00ed2536-3d80-4f07-8851-4f49f1606498 (Autodesk Fusion 360 design; units mm, degrees)
Autodesk Fusion 360 part; units mm, degrees
sketch "Sketch1" plane through (0, 0, 0) normal (0, 0, 1) x (1, 0, 0)
  circle A0 centre (0, 0) radius 7.9375
  circle A1 centre (0, 0) radius 11.1125
  dimension "d1" = 15.875
  dimension "d2" = 22.225
  measures "d1" diameter of A0
  measures "d2" diameter of A1
extrude "Extrude1" add sketch "Sketch1" along normal blind 31.75
sketch "Sketch2" plane through (0, 0, 0) normal (0, 0, -1) x (-1, 0, 0)
  circle A0 centre (0, 0) radius 11.1125
  circle A1 centre (0, 0) radius 14.2875
  circle A2 centre (0, 0) radius 7.9375
  dimension "d5" = 28.575
  measures "d5" diameter of A1
extrude "Extrude2" add sketch "Sketch2" against normal blind 3.175 contours A1
equation "d1 = Shaft_ID"
equation "d2 = Housing_ID"
equation "d3 = Length"
equation "d5 = Flange_OD"
equation "d6 = FlangeT"
equation "Shaft_ID = ( 5 / 8 ) * 1 in"
equation "Housing_ID = ( 7 / 8 ) * 1 in"
equation "FlangeT = ( -1 / 8 ) * 1 in"
equation "Length = 1 1/4\""
equation "Flange_OD = 1 1/8\""
